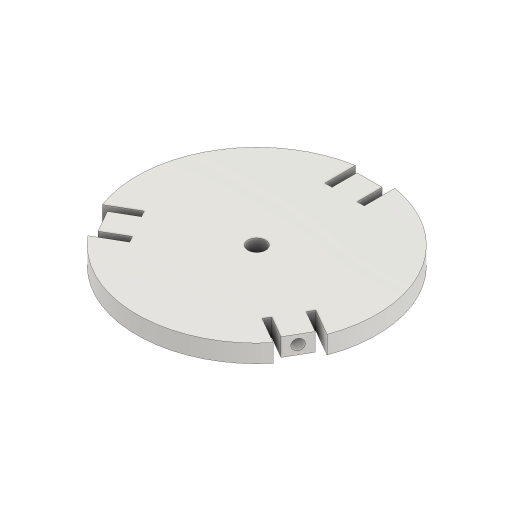
# Autodesk Inventor part: Engine bulkhead
Saved by Autodesk Inventor 2024 (Build 280153000, 153)
## iProperties
Created: 2023-12-30
Part Number: Engine bulkhead
Material: Steel AISI 1006 85 HR
Document SubType Name: Modeling
Designer: Jamie
Density: 7.872 g/cm^3
Appearance: Steel
Author: Jamie
Autodesk Inventor part; units mm, degrees
ref_plane "XZ Plane" through (0, 0, 0) normal (0, 1, 0) x (-1, 0, 0)
ref_plane "XY Plane" through (0, 0, 0) normal (0, 0, 1) x (1, 0, 0)
sketch "Sketch1" plane through (0, 0, 0) normal (0, 1, 0) x (-1, 0, 0)
  circle A0 centre (0, 0) radius 33.5
  dimension "d0" = 67
  constraints: 1 centre point, 1 coincident
  measures "d0" diameter of A0
extrude "Extrusion1" add sketch "Sketch1" along normal blind 5
ref_plane "Work Plane1" through (33.5, 0, 0) normal (1, 0, 0) x (0, 1, 0)
sketch "Sketch3" plane through (0, 0, 0) normal (0, -1, 0) x (1, 0, 0)
  point P0 (0, 0)
  point P1 (0, 0)
  constraints: 1 coincident
hole "Hole2" at (0, 0, 0) direction (0, 1, 0) diameter 5 depth 8 tip angle 118
sketch "Sketch4" plane through (0, 5, 0) normal (0, 1, 0) x (1, 0, 0)
  line L0 (-5.5, 33.0454) -> (5.5, 33.0454) construction
  line L1 (-5.5, 33.0454) -> (-5.5, 24.5)
  line L2 (-5.5, 24.5) -> (-3.5, 24.5)
  line L3 (-3.5, 24.5) -> (-3.5, 31.5)
  line L4 (-3.5, 31.5) -> (3.5, 31.5)
  line L5 (3.5, 31.5) -> (3.5, 24.5)
  line L6 (3.5, 24.5) -> (5.5, 24.5)
  line L7 (5.5, 24.5) -> (5.5, 33.0454)
  circle A0 centre (0, 0) radius 2
  arc A1 (5.5, 33.0454) -> (-5.5, 33.0454) centre (0, 0) ccw
  line L8 (5.5, 33.0454) -> (0, 0) construction
  line L9 (0, 0) -> (0, 33.5) construction
  line L10 (5.5, 24.5) -> (0, 0) construction
  line L11 (8.8419, 25.8873) -> (0, -15.7106) construction
  line L12 (8.8419, 25.8873) -> (8.4261, 23.931) construction
  circle A2 centre (0, 0) radius 33.5 projected
  point P0 (0, 31.5)
  dimension "d22" = 11
  dimension "d23" = 2
  dimension "d24" = 2
  dimension "d25" = 9
  dimension "d26" = 2
  dimension "d28" = 2
  dimension "d29" = 0
  dimension "d31" = 12
  dimension "d35" = 33.5
  constraints: 26 end point, 5 perpendicular, 3 point on circle, 3 point on line, 2 centre point, 2 coincident, 1 concentric, 1 horizontal, 1 midpoint, 1 vertical
  measures "d22" distance of L1.start L7.end
  measures "d23" distance between parallel lines of L3 L1
  measures "d24" distance between parallel lines of L7 L5
  measures "d25" distance from line of L9.end L6
  measures "d26" distance of L9.end point (0, 31.5)
  measures "d28" distance of L12.start L12.end
  measures "d29" horizontal distance of point (0, 0) L11.end
  measures "d31" angle of L9 L11
  measures "d35" distance of point (0, 0) L1.start
extrude "Extrusion2" cut sketch "Sketch4" against normal blind 10 contours A1 L7 L6 L5 L4 L3 L2 L1
sketch "Sketch5" plane through (3.5, 5, -31.5) normal (0, 0, -1) x (-1, 0, 0)
  line L0 (0, 0) -> (7, 0) projected
  point P0 (3.5, -5)
  point P1 (3.5, -2.5)
  dimension "d36" = 2.5
  measures "d36" distance from line of point (3.5, -2.5) L0
hole "Hole3" at (0, 2.5, -31.5) direction (0, 0, 1) diameter 3 depth 16 tip angle 118
pattern_circular "Circular Pattern2" count 3 over 360 about axis through (0, 0, 0) along (0, 1, 0) of "Hole3", "Extrusion2"
body "Solid1"
